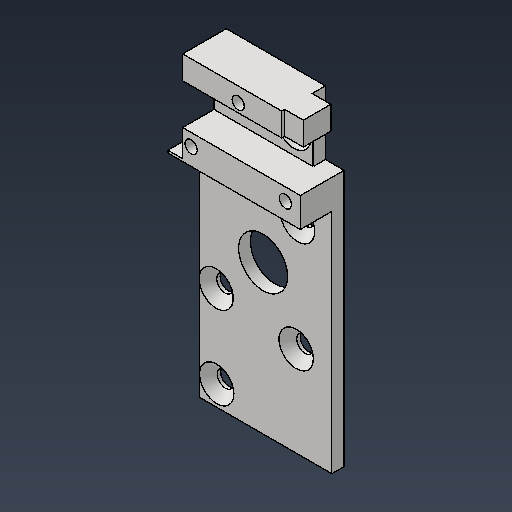
# Autodesk Inventor part: RightGearboxCover
Saved by Autodesk Inventor 2026.2 (Build 302298010, 298A)
## iProperties
Created: 2026-04-04
Part Number: RightGearboxCover
Material: Generic
Document SubType Name: Modeling
Designer: szymo
Density: 1 g/cm^3
Appearance: Default
Author: szymo
Autodesk Inventor part; units mm, degrees
ref_plane "YZ Plane" through (0, 0, 0) normal (1, 0, 0) x (0, 1, 0)
ref_plane "XZ Plane" through (0, 0, 0) normal (0, 1, 0) x (-1, 0, 0)
ref_plane "XY Plane" through (0, 0, 0) normal (0, 0, 1) x (1, 0, 0)
ref_plane "Work Plane1" through (0, -65.2958, -0.3) normal (0, 0, 1) x (1, 0, 0)
ref_plane "Work Plane4" through (0.0409, -65.2958, -0.1) normal (0, 0, 1) x (1, 0, 0)
sketch "Sketch1" plane through (0, 0, 0) normal (0, 0, 1) x (1, 0, 0)
  circle A0 centre (13, -35.0012) radius 5
  circle A1 centre (13, -35.0012) radius 5.6
  circle A2 centre (8.3716, -9.3577) radius 1.0564
  circle A3 centre (20.6284, -19.6423) radius 1.0564 construction
  circle A4 centre (14.5, -14.5) radius 5 construction
  circle A5 centre (14.5, -14.5) radius 13.85 construction
  circle A6 centre (14.5, -14.5) radius 14.5 construction
  circle A7 centre (14.5, -55.2958) radius 14.5 construction
  circle A8 centre (14.5, -55.2958) radius 13.85 construction
  line L0 (27, 0) -> (0, 0)
  line L1 (0, 0) -> (0, -65.2958)
  line L2 (0, -65.2958) -> (27, -65.2958)
  line L3 (27, -65.2958) -> (27, 0)
  line L4 (1, -17) -> (1, -13.9)
  line L5 (1, -13.9) -> (0, -13.9)
  line L6 (0, -13.9) -> (0, -18)
  line L7 (0, -18) -> (2.4477, -18)
  arc A9 (2.5, -17.9298) -> (2.4477, -18) centre (9.2084, -22.9852) ccw
  line L8 (2.5, -17.9298) -> (2.5, -17)
  line L9 (2.5, -17) -> (1, -17)
  line L10 (3, 0) -> (3, -18.5)
  line L11 (3, -18.5) -> (0, -18.5)
  line L12 (3, -3) -> (27, -3)
  line L13 (27, -13) -> (3, -13)
  line L14 (23.2, 0) -> (23.2, -39.2749)
  arc A10 (20.6322, -38.1335) -> (22.0597, -38.1763) centre (21.5245, -32.1971) ccw
  arc A11 (22.0597, -38.1763) -> (22.2135, -37.6978) centre (13, -35.0012) ccw
  arc A12 (22.2135, -37.6978) -> (21.0283, -36.901) centre (18.2955, -42.246) ccw
  arc A13 (21.0283, -36.901) -> (21.1167, -36.4782) centre (13, -35.0012) ccw
  arc A14 (21.1167, -36.4782) -> (22.5219, -36.2233) centre (20.7552, -30.4861) ccw
  arc A15 (22.5219, -36.2233) -> (22.5728, -35.7233) centre (13, -35.0012) ccw
  arc A16 (22.5728, -35.7233) -> (21.2478, -35.1903) centre (19.6861, -40.9866) ccw
  arc A17 (21.2478, -35.1903) -> (21.2464, -34.7584) centre (13, -35.0012) ccw
  arc A18 (21.2464, -34.7584) -> (22.5679, -34.2168) centre (19.647, -28.9724) ccw
  arc A19 (22.5679, -34.2168) -> (22.5137, -33.7172) centre (13, -35.0012) ccw
  arc A20 (22.5137, -33.7172) -> (21.1069, -33.4714) centre (20.7844, -39.4657) ccw
  arc A21 (21.1069, -33.4714) -> (21.0157, -33.0492) centre (13, -35.0012) ccw
  arc A22 (21.0157, -33.0492) -> (22.1957, -32.2447) centre (18.2483, -27.7221) ccw
  arc A23 (22.1957, -32.2447) -> (22.0389, -31.7672) centre (13, -35.0012) ccw
  arc A24 (22.0389, -31.7672) -> (20.6117, -31.8193) centre (21.5425, -37.7497) ccw
  arc A25 (20.6117, -31.8193) -> (20.4347, -31.4253) centre (13, -35.0012) ccw
  arc A26 (20.4347, -31.4253) -> (21.4217, -30.393) centre (16.6202, -26.79) ccw
  arc A27 (21.4217, -30.393) -> (21.169, -29.9586) centre (13, -35.0012) ccw
  arc A28 (21.169, -29.9586) -> (19.7838, -30.3062) centre (21.9273, -35.9136) ccw
  arc A29 (19.7838, -30.3062) -> (19.5288, -29.9576) centre (13, -35.0012) ccw
  arc A30 (19.5288, -29.9576) -> (20.2796, -28.7428) centre (14.8338, -26.2168) ccw
  arc A31 (20.2796, -28.7428) -> (19.9421, -28.3704) centre (13, -35.0012) ccw
  arc A32 (19.9421, -28.3704) -> (18.6594, -28.9984) centre (21.9219, -34.0375) ccw
  arc A33 (18.6594, -28.9984) -> (18.3375, -28.7104) centre (13, -35.0012) ccw
  arc A34 (18.3375, -28.7104) -> (18.8193, -27.366) centre (12.9674, -26.0275) ccw
  arc A35 (18.8193, -27.366) -> (18.4117, -27.0719) centre (13, -35.0012) ccw
  arc A36 (18.4117, -27.0719) -> (17.2877, -27.9529) centre (21.5266, -32.2036) ccw
  arc A37 (17.2877, -27.9529) -> (16.9129, -27.7382) centre (13, -35.0012) ccw
  arc A38 (16.9129, -27.7382) -> (17.1047, -26.323) centre (11.1024, -26.2303) ccw
  arc A39 (17.1047, -26.323) -> (16.6449, -26.12) centre (13, -35.0012) ccw
  arc A40 (16.6449, -26.12) -> (15.7286, -27.2155) centre (20.7586, -30.492) ccw
  arc A41 (15.7286, -27.2155) -> (15.3174, -27.0834) centre (13, -35.0012) ccw
  arc A42 (15.3174, -27.0834) -> (15.2107, -25.6592) centre (9.3203, -26.8165) ccw
  arc A43 (15.2107, -25.6592) -> (14.7187, -25.5563) centre (13, -35.0012) ccw
  arc A44 (14.7187, -25.5563) -> (14.0502, -26.8183) centre (19.6515, -28.9774) ccw
  arc A45 (14.0502, -26.8183) -> (13.6205, -26.7746) centre (13, -35.0012) ccw
  arc A46 (13.6205, -26.7746) -> (13.2201, -25.4037) centre (7.699, -27.7605) ccw
  arc A47 (13.2201, -25.4037) -> (12.7175, -25.4054) centre (13, -35.0012) ccw
  arc A48 (12.7175, -25.4054) -> (12.3259, -26.7788) centre (18.2538, -27.7261) ccw
  arc A49 (12.3259, -26.7788) -> (11.8965, -26.8253) centre (13, -35.0012) ccw
  arc A50 (11.8965, -26.8253) -> (11.2198, -25.5677) centre (6.3094, -29.0208) ccw
  arc A51 (11.2198, -25.5677) -> (10.7286, -25.6738) centre (13, -35.0012) ccw
  arc A52 (10.7286, -25.6738) -> (10.6311, -27.0986) centre (16.6264, -26.7928) ccw
  arc A53 (10.6311, -27.0986) -> (10.2208, -27.2334) centre (13, -35.0012) ccw
  arc A54 (10.2208, -27.2334) -> (9.2974, -26.144) centre (5.2122, -30.5426) ccw
  arc A55 (9.2974, -26.144) -> (8.8389, -26.3499) centre (13, -35.0012) ccw
  arc A56 (8.8389, -26.3499) -> (9.0399, -27.7638) centre (14.8405, -26.2182) ccw
  arc A57 (9.0399, -27.7638) -> (8.6665, -27.981) centre (13, -35.0012) ccw
  arc A58 (8.6665, -27.981) -> (7.5368, -27.1073) centre (4.4554, -32.2592) ccw
  arc A59 (7.5368, -27.1073) -> (7.1311, -27.4041) centre (13, -35.0012) ccw
  arc A60 (7.1311, -27.4041) -> (7.6217, -28.7453) centre (12.9742, -26.0274) ccw
  arc A61 (7.6217, -28.7453) -> (7.3016, -29.0354) centre (13, -35.0012) ccw
  arc A62 (7.3016, -29.0354) -> (6.0149, -28.4157) centre (4.072, -34.0956) ccw
  arc A63 (6.0149, -28.4157) -> (5.6799, -28.7903) centre (13, -35.0012) ccw
  arc A64 (5.6799, -28.7903) -> (6.4385, -30.0002) centre (11.109, -26.2289) ccw
  arc A65 (6.4385, -30.0002) -> (6.1858, -30.3505) centre (13, -35.0012) ccw
  arc A66 (6.1858, -30.3505) -> (4.7984, -30.0119) centre (4.0788, -35.9716) ccw
  arc A67 (4.7984, -30.0119) -> (4.5485, -30.448) centre (13, -35.0012) ccw
  arc A68 (4.5485, -30.448) -> (5.5422, -31.4737) centre (9.3265, -26.8137) ccw
  arc A69 (5.5422, -31.4737) -> (5.3678, -31.8689) centre (13, -35.0012) ccw
  arc A70 (5.3678, -31.8689) -> (3.9403, -31.8261) centre (4.4755, -37.8053) ccw
  arc A71 (3.9403, -31.8261) -> (3.7865, -32.3046) centre (13, -35.0012) ccw
  arc A72 (3.7865, -32.3046) -> (4.9717, -33.1014) centre (7.7045, -27.7564) ccw
  arc A73 (4.9717, -33.1014) -> (4.8833, -33.5242) centre (13, -35.0012) ccw
  arc A74 (4.8833, -33.5242) -> (3.4781, -33.7791) centre (5.2448, -39.5163) ccw
  arc A75 (3.4781, -33.7791) -> (3.4272, -34.2791) centre (13, -35.0012) ccw
  arc A76 (3.4272, -34.2791) -> (4.7522, -34.8121) centre (6.3139, -29.0157) ccw
  arc A77 (4.7522, -34.8121) -> (4.7536, -35.244) centre (13, -35.0012) ccw
  arc A78 (4.7536, -35.244) -> (3.4321, -35.7855) centre (6.353, -41.03) ccw
  arc A79 (3.4321, -35.7855) -> (3.4863, -36.2852) centre (13, -35.0012) ccw
  arc A80 (3.4863, -36.2852) -> (4.8931, -36.531) centre (5.2156, -30.5367) ccw
  arc A81 (4.8931, -36.531) -> (4.9843, -36.9532) centre (13, -35.0012) ccw
  arc A82 (4.9843, -36.9532) -> (3.8043, -37.7577) centre (7.7517, -42.2803) ccw
  arc A83 (3.8043, -37.7577) -> (3.9611, -38.2352) centre (13, -35.0012) ccw
  arc A84 (3.9611, -38.2352) -> (5.3883, -38.1831) centre (4.4575, -32.2527) ccw
  arc A85 (5.3883, -38.1831) -> (5.5653, -38.5771) centre (13, -35.0012) ccw
  arc A86 (5.5653, -38.5771) -> (4.5783, -39.6094) centre (9.3798, -43.2124) ccw
  arc A87 (4.5783, -39.6094) -> (4.831, -40.0438) centre (13, -35.0012) ccw
  arc A88 (4.831, -40.0438) -> (6.2162, -39.6962) centre (4.0727, -34.0888) ccw
  arc A89 (6.2162, -39.6962) -> (6.4712, -40.0448) centre (13, -35.0012) ccw
  arc A90 (6.4712, -40.0448) -> (5.7204, -41.2596) centre (11.1662, -43.7856) ccw
  arc A91 (5.7204, -41.2596) -> (6.0579, -41.632) centre (13, -35.0012) ccw
  arc A92 (6.0579, -41.632) -> (7.3406, -41.004) centre (4.0781, -35.9649) ccw
  arc A93 (7.3406, -41.004) -> (7.6625, -41.292) centre (13, -35.0012) ccw
  arc A94 (7.6625, -41.292) -> (7.1807, -42.6364) centre (13.0326, -43.9749) ccw
  arc A95 (7.1807, -42.6364) -> (7.5883, -42.9305) centre (13, -35.0012) ccw
  arc A96 (7.5883, -42.9305) -> (8.7123, -42.0495) centre (4.4734, -37.7988) ccw
  arc A97 (8.7123, -42.0495) -> (9.0871, -42.2642) centre (13, -35.0012) ccw
  arc A98 (9.0871, -42.2642) -> (8.8953, -43.6794) centre (14.8976, -43.7721) ccw
  arc A99 (8.8953, -43.6794) -> (9.3551, -43.8824) centre (13, -35.0012) ccw
  arc A100 (9.3551, -43.8824) -> (10.2714, -42.7869) centre (5.2414, -39.5104) ccw
  arc A101 (10.2714, -42.7869) -> (10.6826, -42.919) centre (13, -35.0012) ccw
  arc A102 (10.6826, -42.919) -> (10.7893, -44.3432) centre (16.6797, -43.1859) ccw
  arc A103 (10.7893, -44.3432) -> (11.2813, -44.4461) centre (13, -35.0012) ccw
  arc A104 (11.2813, -44.4461) -> (11.9498, -43.1841) centre (6.3485, -41.025) ccw
  arc A105 (11.9498, -43.1841) -> (12.3795, -43.2278) centre (13, -35.0012) ccw
  arc A106 (12.3795, -43.2278) -> (12.7799, -44.5987) centre (18.301, -42.2419) ccw
  arc A107 (12.7799, -44.5987) -> (13.2825, -44.597) centre (13, -35.0012) ccw
  arc A108 (13.2825, -44.597) -> (13.6741, -43.2236) centre (7.7462, -42.2763) ccw
  arc A109 (13.6741, -43.2236) -> (14.1035, -43.1771) centre (13, -35.0012) ccw
  arc A110 (14.1035, -43.1771) -> (14.7802, -44.4347) centre (19.6906, -40.9816) ccw
  arc A111 (14.7802, -44.4347) -> (15.2714, -44.3286) centre (13, -35.0012) ccw
  arc A112 (15.2714, -44.3286) -> (15.3689, -42.9038) centre (9.3736, -43.2096) ccw
  arc A113 (15.3689, -42.9038) -> (15.7792, -42.769) centre (13, -35.0012) ccw
  arc A114 (15.7792, -42.769) -> (16.7026, -43.8584) centre (20.7878, -39.4598) ccw
  arc A115 (16.7026, -43.8584) -> (17.1611, -43.6525) centre (13, -35.0012) ccw
  arc A116 (17.1611, -43.6525) -> (16.9601, -42.2386) centre (11.1595, -43.7842) ccw
  arc A117 (16.9601, -42.2386) -> (17.3335, -42.0214) centre (13, -35.0012) ccw
  arc A118 (17.3335, -42.0214) -> (18.4632, -42.8951) centre (21.5446, -37.7432) ccw
  arc A119 (18.4632, -42.8951) -> (18.8689, -42.5983) centre (13, -35.0012) ccw
  arc A120 (18.8689, -42.5983) -> (18.3783, -41.2571) centre (13.0258, -43.975) ccw
  arc A121 (18.3783, -41.2571) -> (18.6984, -40.967) centre (13, -35.0012) ccw
  arc A122 (18.6984, -40.967) -> (19.9851, -41.5867) centre (21.928, -35.9068) ccw
  arc A123 (19.9851, -41.5867) -> (20.3201, -41.2121) centre (13, -35.0012) ccw
  arc A124 (20.3201, -41.2121) -> (19.5615, -40.0022) centre (14.891, -43.7735) ccw
  arc A125 (19.5615, -40.0022) -> (19.8142, -39.6519) centre (13, -35.0012) ccw
  arc A126 (19.8142, -39.6519) -> (21.2016, -39.9905) centre (21.9212, -34.0308) ccw
  arc A127 (21.2016, -39.9905) -> (21.4515, -39.5544) centre (13, -35.0012) ccw
  arc A128 (21.4515, -39.5544) -> (20.4578, -38.5287) centre (16.6735, -43.1886) ccw
  arc A129 (20.4578, -38.5287) -> (20.6322, -38.1335) centre (13, -35.0012) ccw
  circle A130 centre (13, -35.0012) radius 9.6 construction
  point P0 (0, 0)
  point P1 (23.2, -13)
  point P2 (23.2, -3)
extrude "Extrusion1" add sketch "Sketch1" against normal up to surface (0.1 mm away) contours A2 | L14 L12 L10 L0 | L14 L13 L10 L12 | L3 L2 L1 L11 L10 L13 | A129 A128 A127 A126 A125 A124 A123 A122 A121 A120 A119 A118 A117 A116 A115 A114 A113 A112 A111 A110 A109 A108 A107 A106 A105 A104 A103 A102 A101 A100 A99 A98 A97 A96 A95 A94 A93 A92 A91 A90 A89 A88 A87 A86 A85 A84 A83 A82 A81 A80 A79 A78 A77 A76 A75 A74 A73 A72 A71 A70 A69 A68 A67 A66 A65 A64 A63 A62 A61 A60 A59 A58 A57 A56 A55 A54 A53 A52 A51 A50 A49 A48 A47 A46 A45 A44 A43 A42 A41 A40 A39 A38 A37 A36 A35 A34 A33 A32 A31 A30 A29 A28 A27 A26 A25 A24 A23 A22 A21 A20 A19 A18 A17 A16 A15 A14 A13 A12 A11 A10
ref_plane "Work Plane2" through (8.0794, -39.9218, 2.4) normal (0, 0, 1) x (0.9996763, -0.0254413, 0)
extrude "Extrusion2" add sketch "Sketch1" along normal up to surface (2.4 mm away) contours A1 | A2 | L14 L12 L10 L0 | L14 L13 L10 L12 | L3 L2 L1 L11 L10 L13 | A129 A128 A127 A126 A125 A124 A123 A122 A121 A120 A119 A118 A117 A116 A115 A114 A113 A112 A111 A110 A109 A108 A107 A106 A105 A104 A103 A102 A101 A100 A99 A98 A97 A96 A95 A94 A93 A92 A91 A90 A89 A88 A87 A86 A85 A84 A83 A82 A81 A80 A79 A78 A77 A76 A75 A74 A73 A72 A71 A70 A69 A68 A67 A66 A65 A64 A63 A62 A61 A60 A59 A58 A57 A56 A55 A54 A53 A52 A51 A50 A49 A48 A47 A46 A45 A44 A43 A42 A41 A40 A39 A38 A37 A36 A35 A34 A33 A32 A31 A30 A29 A28 A27 A26 A25 A24 A23 A22 A21 A20 A19 A18 A17 A16 A15 A14 A13 A12 A11 A10
sketch "Sketch2" plane through (27, -65.2958, -0.1) normal (0, 0, -1) x (-1, 0, 0)
  circle A0 centre (12.5, 50.7958) radius 1.15 projected
  circle A1 centre (12.5, 50.7958) radius 1.65
  circle A2 centre (17.7916, 42.3106) radius 3 projected
  point P0 (27, 65.2958)
  dimension "d9" = 0.5
  constraints: 1 centre point
  measures "d9" radial gap between concentric circles of A0 A1
extrude "Extrusion3" cut sketch "Sketch2" against normal blind 2 contours A0 | A1
ref_plane "Work Plane3" through (1, -19, 8.2) normal (0, 0, -1) x (0, 1, 0)
sketch "Sketch4" plane through (0, -65.2958, 2.4) normal (0, 0, 1) x (1, 0, 0)
  circle A0 centre (14.325, 62.2958) radius 0.75 projected
  circle A1 centre (4.725, 49.7467) radius 0.75 projected
  circle A2 centre (23.925, 49.7467) radius 0.75 projected
  line L0 (23.7668, 46.2958) -> (4.8832, 46.2958) projected
  arc A3 (4.8832, 46.2958) -> (4.8444, 46.2989) centre (4.825, 45.7992) ccw projected
  arc A4 (1, 50.2958) -> (4.8444, 46.2989) centre (5, 50.2958) ccw projected
  line L1 (1, 60.2958) -> (1, 50.2958) projected
  arc A5 (6, 65.2958) -> (1, 60.2958) centre (6, 60.2958) ccw projected
  line L2 (22.65, 65.2958) -> (6, 65.2958) projected
  arc A6 (27.65, 60.2958) -> (22.65, 65.2958) centre (22.65, 60.2958) ccw projected
  line L3 (27.65, 50.2958) -> (27.65, 60.2958) projected
  arc A7 (23.8056, 46.2989) -> (27.65, 50.2958) centre (23.65, 50.2958) ccw projected
  arc A8 (23.8056, 46.2989) -> (23.7668, 46.2958) centre (23.825, 45.7992) ccw projected
  line L4 (23.2, 65.2958) -> (23.2, 52.2958) projected
  line L5 (23.2, 52.2958) -> (3, 52.2958)
  line L6 (3, 46.7958) -> (3, 65.2958) projected
  line L7 (27, 52.2958) -> (27, 0) projected
  line L8 (27, 46.2958) -> (0, 46.2958)
  line L9 (0, 0) -> (0, 46.7958) projected
  line L10 (23.2, 60.5458) -> (3, 60.5458)
  line L11 (3, 65.2958) -> (23.2, 65.2958) projected
  line L12 (3, 65.2958) -> (23.2, 65.2958) projected
  line L13 (0, 46.7958) -> (3, 46.7958) projected
  line L14 (0, 46.7958) -> (3, 46.7958) projected
  line L15 (27, 52.2958) -> (27, 0) projected
  line L16 (27, 52.2958) -> (27, 0) projected
  line L17 (27, 62.2958) -> (23.8, 62.2958) projected
  line L18 (27, 62.2958) -> (23.8, 62.2958) projected
  line L19 (23.2, 52.2958) -> (27, 52.2958) projected
  line L20 (23.2, 52.2958) -> (27, 52.2958) projected
  line L21 (23.8, 62.2958) -> (23.8, 65.2958)
  point P0 (0, 65.2958)
  point P1 (27, 52.2958)
  point P2 (3, 46.7958)
  point P3 (0, 46.7958)
  point P4 (4.8832, 46.2958)
  point P5 (27, 65.2958)
  point P6 (22.65, 65.2958)
  point P7 (3, 65.2958)
  point P8 (23.8, 62.2958)
  point P9 (27, 62.2958)
  point P10 (23.8, 62.2958)
  point P11 (23.2, 65.2958)
  dimension "d15" = 1
  constraints: 6 end point, 5 point on line, 1 collinear, 1 horizontal, 1 parallel, 1 perpendicular, 5 other
  measures "d15" distance edge to line of A0 L10
extrude "Extrusion4" add sketch "Sketch4" along normal blind 6.4 contours A0 | A1 | A2 | L0 A3 A4 L6 L5 L19 L7 A7 A8 | A8 A7 L7 L8 | L8 L9 L13 L6 A4 A3 | L6 A5 L2 A6 L4 L10 | L6 L11 A5 | A6 L11 L4
sketch "Sketch5" plane through (27, -65.2958, -0.1) normal (0, 0, -1) x (-1, 0, 0)
  circle A0 centre (12.675, 62.2958) radius 0.75 projected
  circle A1 centre (22.275, 49.7467) radius 0.75 projected
  circle A2 centre (3.075, 49.7467) radius 0.75 projected
  line L0 (3.2332, 46.2958) -> (22.1168, 46.2958) projected
  arc A3 (22.1556, 46.2989) -> (22.1168, 46.2958) centre (22.175, 45.7992) ccw projected
  arc A4 (22.1556, 46.2989) -> (26, 50.2958) centre (22, 50.2958) ccw projected
  line L1 (26, 60.2958) -> (26, 50.2958) projected
  arc A5 (26, 60.2958) -> (21, 65.2958) centre (21, 60.2958) ccw projected
  line L2 (4.35, 65.2958) -> (21, 65.2958) projected
  arc A6 (4.35, 65.2958) -> (-0.65, 60.2958) centre (4.35, 60.2958) ccw projected
  line L3 (-0.65, 50.2958) -> (-0.65, 60.2958) projected
  arc A7 (-0.65, 50.2958) -> (3.1944, 46.2989) centre (3.35, 50.2958) ccw projected
  arc A8 (3.2332, 46.2958) -> (3.1944, 46.2989) centre (3.175, 45.7992) ccw projected
  point P0 (27, 65.2958)
hole "Hole1" at (23.925, -15.5491, -0.1) at (14.325, -3, -0.1) at (4.725, -15.5491, -0.1) direction (0, 0, 1) diameter 3 depth 4.5 counterbore diameter 3.5 counterbore depth 0.5
hole "Hole2" at (23.925, -15.5491, -0.1) at (14.325, -3, -0.1) at (4.725, -15.5491, -0.1) direction (0, 0, 1) diameter 2.5 end through all
hole "Hole3" at (9.2084, -22.9852, -0.1) direction (0, 0, 1) diameter 2.5 depth 2
sketch "Sketch6" plane through (0, -65.2958, 2.4) normal (0, 0, 1) x (1, 0, 0)
  circle A0 centre (19.2409, 57.0458) radius 2 projected
  circle A1 centre (19.7409, 18.3957) radius 2.25 projected
  circle A2 centre (3.5409, 4.125) radius 2 projected
  circle A3 centre (3.4336, 20.9055) radius 2 projected
  circle A4 centre (3.4336, 20.9055) radius 2.25 projected
  circle A5 centre (20.0127, 40.9491) radius 2.25 projected
  point P0 (0, 65.2958)
  point P1 (19.7, 61.7958)
hole "Hole4" at (19.2409, -8.25, 2.4) at (19.7409, -46.9002, 2.4) at (3.5409, -61.1709, 2.4) at (3.4336, -44.3904, 2.4) at (20.0127, -24.3467, 2.4) direction (0, 0, -1) diameter 3.4 depth 7 countersink diameter 7 countersink angle 90 clearance for "Countersunk Flat Head Screw ISO 2009/7046" size "M3" standard "ISO"
sketch "Sketch7" plane through (3, 0, -0.1) normal (0, 1, 0) x (1, 0, 0)
  line L0 (20.2, 0) -> (24, 0) projected
  line L1 (20.2, 0) -> (20.2, -2.5) projected
  line L2 (0, -2.5) -> (20.2, -2.5) projected
  line L3 (0, -2.5) -> (0, -8.9) projected
  line L4 (24, 0) -> (24, -8.9) projected
  line L5 (20.2, 10.5) -> (20.2, -2.6) projected
  line L6 (20.2, -2.6) -> (21, -2.6) projected
  line L7 (21, 10.5) -> (21, -2.6) projected
  line L8 (20.2, 10.5) -> (21, 10.5) projected
  line L9 (24, 0) -> (24, -8.3) projected
  line L10 (20.2, -8.3) -> (24, -8.3)
  line L11 (24, -8.3) -> (24, -2.7)
  line L12 (24, -2.7) -> (20.2, -2.7)
  line L13 (20.2, -2.7) -> (20.2, -8.3)
  line L14 (24, -8.9) -> (0, -8.9) projected
  point P0 (-3, -0.1)
  point P1 (24, -2.7)
  dimension "d47" = 0.1
  dimension "d48" = 0
  constraints: 8 end point, 2 parallel, 1 horizontal, 1 perpendicular, 1 point on line
  measures "d47" distance between parallel lines of L6 L12
  measures "d48" distance between parallel lines of L1 L13
extrude "Extrusion5" add sketch "Sketch7" against normal up to surface (4.75 mm away) contours L4 L10 L13 L12
body "Solid1"
